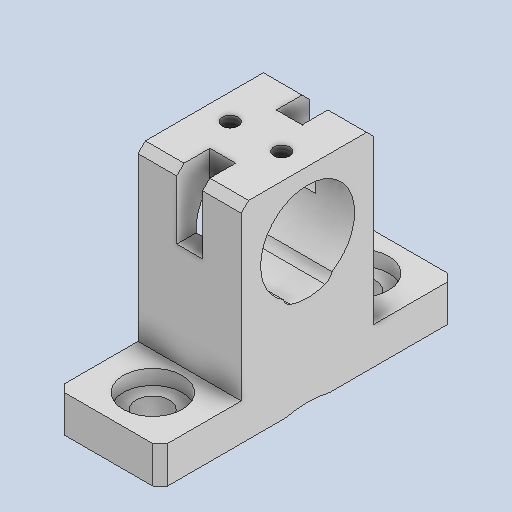
# Autodesk Inventor part: ADAPTER_collimator-BH19.05-D12.7
Saved by Autodesk Inventor 2024.2 (Build 282272000, 272)
## iProperties
Created: 2020-10-22
Part Number: ADAPTER_collimator-BH19.05-D12.7
Material: Generic
Document SubType Name: Modeling
Designer: qiti1
Density: 1 g/cm^3
Appearance: Default
ItemSpecifications: {"_id":"603fbb7ae0b54a000914fb10","finish":"543ef1f380da5b0c476373c1","finish_location":null,"material":"5515e170db035c20ce34af9a","process_initialism":null,"quotes":null,"current_quote":null,"quantity_ordered":1,"features":null,"hardware":null,"threading":null,"part_markings":[],"surface_roughness":null,"tolerance":null,"weld_quantity":null,"Notes":"","certifications":[],"part":null,"revision_num":0,"last_history":null,"inspection_requirement_details":{"inspection_requirement":"std","customer_data_sheet":null},"feedback":null}
Author: qiti1
Autodesk Inventor part; units mm, degrees
note: some values were not read from the file. Chosen so that the rebuilt part matches the saved one: direction of "Hole3".
ref_plane "YZ Plane" through (0, 0, 0) normal (1, 0, 0) x (0, 1, 0)
ref_plane "XZ Plane" through (0, 0, 0) normal (0, 1, 0) x (-1, 0, 0)
ref_plane "XY Plane" through (0, 0, 0) normal (0, 0, 1) x (1, 0, 0)
sketch "Sketch1" plane through (0, 0, 0) normal (0, 1, 0) x (-1, 0, 0)
  line L0 (7, 9) -> (-7, 9)
  line L1 (-7, 9) -> (-7, -9)
  line L2 (-7, -9) -> (7, -9)
  line L3 (7, -9) -> (7, 9)
  line L4 (7, 9) -> (-7, -9) construction
  line L5 (-7, 9) -> (7, -9) construction
  point P0 (0, 0)
  dimension "POST_WIDTH" = 18
  dimension "POST_LENGTH" = 14
  constraints: 12 end point, 2 midpoint, 2 parallel, 1 horizontal, 1 perpendicular
  measures "POST_WIDTH" distance of L2.end L0.start
  measures "POST_LENGTH" distance of L1.end L2.end
extrude "Extrusion1" add sketch "Sketch1" along normal blind 28.05
sketch "Sketch2" plane through (0, 0, 0) normal (0, -1, 0) x (1, 0, 0)
  line L0 (-7, -20) -> (7, -20)
  line L1 (7, -20) -> (7, 20)
  line L2 (7, 20) -> (-7, 20)
  line L3 (-7, 20) -> (-7, -20)
  line L4 (-7, -20) -> (7, 20) construction
  line L5 (7, -20) -> (-7, 20) construction
  line L6 (-7, -9) -> (-7, 9) projected
  line L7 (-7, 9) -> (7, 9) projected
  point P0 (0, 0)
  dimension "d4" = 0
  dimension "d5" = 11
  constraints: 12 end point, 2 midpoint, 2 parallel, 1 horizontal, 1 perpendicular
  measures "d4" distance between parallel lines of L6 L3
  measures "d5" distance between parallel lines of L2 L7
extrude "Extrusion2" add sketch "Sketch2" against normal blind 5
sketch "Sketch3" plane through (0, 5, 0) normal (0, 1, 0) x (1, 0, 0)
  line L0 (-7, 20) -> (7, 20) projected
  line L1 (0, 20) -> (0, -20)
  line L2 (7, -20) -> (-7, -20) projected
  line L3 (7, -9) -> (7, 9) projected
  line L4 (7, 0) -> (-7, 0)
  line L5 (-7, 20) -> (-7, -20) projected
  point P0 (0, 0)
  point P1 (0, -14)
  point P2 (0, 14)
  dimension "d15" = 0
  dimension "d16" = 6
  constraints: 4 end point, 4 midpoint, 1 symmetric about line
  measures "d15" distance from line of L1 point (0, -14)
  measures "d16" distance from line of L2 point (0, -14)
hole "Hole1" at (0, 5, 14) at (0, 5, -14) direction (0, -1, 0) diameter 4.5 end through all counterbore diameter 8 counterbore depth 2 clearance for "Socket Head Cap Screw" size "#8" standard "Ansi Unified Screw Threads"
chamfer "Chamfer2" distance 1 angle 45 2 edges at (0, 28.05, 9) (0, 28.05, -9)
sketch "Sketch8" plane through (7, 5, -9) normal (1, 0, 0) x (0, 0, -1)
  circle A0 centre (-9, 14.4933) radius 6.375
  circle A1 centre (-9, 14.4933) radius 6.883
  circle A2 centre (-10.8329, 9.4575) radius 1.524
  line L0 (-9, 14.4933) -> (-9, 7.6103)
  circle A3 centre (-7.1671, 9.4575) radius 1.524
  line L1 (-9, 14.4933) -> (-10.8329, 9.4575)
  line L2 (-18, 0) -> (-18, 22.05) projected
  line L3 (-17, 23.05) -> (-1, 23.05) projected
  circle A4 centre (-9, 14.05) radius 6
  line L4 (11, -5) -> (-29, -5) projected
  point P0 (-9, -5)
  point P1 (-6.6459, 8.0254)
  point P2 (-8.0195, 8.1942)
  point P3 (-12.2979, 9.0376)
  point P4 (-11.3541, 8.0254)
  point P5 (-5.7021, 9.0376)
  point P6 (-9.9805, 8.1942)
  dimension "d95" = 12
  dimension "HOLE_SIZE" = 12.75
  dimension "THREE_POINT_SIZE" = 13.766
  dimension "d51" = 3.048
  dimension "d52" = 20
  dimension "d55" = 9
  dimension "d96" = 19.05
  constraints: 4 end point, 1 centre point, 1 coincident, 1 point on line, 1 symmetric about line, 1 vertical, 14 other
  measures "d51" diameter of A2
  measures "d52" angle of L0 L1
  measures "d55" distance from line of L2 point (-9, 14.493)
  measures "d96" distance from line of L4 point (-9, 14.05)
extrude "Extrusion6" cut sketch "Sketch8" against normal up to surface (14 mm away) contours A0 A4 | A2 A0 | A4 A3 A0 L0 L1 A2 | A4 A2 | A0 A2 A4 | A4 A3 A0 | A0 A3 | A3 A4 | A2 L1 L0 A0 | A0 L0 A4 A2 | A2 A4 L0 A1 | A3 A4 L0 A0 | A1 L0 A4 A3
sketch "Sketch9" plane through (0, 28.05, 0) normal (0, 1, 0) x (1, 0, 0)
  line L0 (-7, 8) -> (-7, -8) projected
  line L1 (-7, -9) -> (7, -9) projected
  line L2 (7, -8) -> (7, 8) projected
  point P0 (0, 0)
  point P1 (-3.5, 0)
  point P2 (3.5, 0)
  dimension "d64" = 3.5
  dimension "d65" = 9
  dimension "d94" = 3.5
  measures "d64" distance from line of L0 point (-3.5, 0)
  measures "d65" distance from line of L1 point (-3.5, 0)
  measures "d94" distance from line of point (3.5, 0) L2
hole "Hole3" at (-3.5, 28.05, 0) at (3.5, 28.05, 0) direction (0, -1, 0) diameter 2.1565 end up to surface thread size "4-40 UNC" class "2B" standard "ANSI Unified Screw Threads"
chamfer "Chamfer3" distance 1 angle 45 4 edges at (7, 2.5, 20) (-7, 2.5, 20) (7, 2.5, -20) (-7, 2.5, -20)
sketch "Sketch10" plane through (0, 28.05, 0) normal (0, 1, 0) x (1, 0, 0)
  line L0 (-7, -9) -> (7, -9) projected
  line L1 (-1.75, -9) -> (1.75, -9)
  line L2 (1.75, -9) -> (1.75, -4.5)
  line L3 (1.75, -4.5) -> (-1.75, -4.5)
  line L4 (-1.75, -4.5) -> (-1.75, -9)
  line L5 (7, 9) -> (-7, 9) projected
  line L6 (-9.8, 0) -> (9.8, 0) projected
  line L7 (-1.75, 9) -> (1.75, 9)
  line L8 (1.75, 9) -> (1.75, 4.5)
  line L9 (1.75, 4.5) -> (-1.75, 4.5)
  line L10 (-1.75, 4.5) -> (-1.75, 9)
  point P0 (0, 0)
  point P1 (1.75, 5.6664)
  point P2 (1.75, 9)
  dimension "d71" = 4.5
  dimension "d72" = 3.5
  dimension "d73" = 1.75
  constraints: 16 end point, 4 point on line, 3 symmetric about line, 2 parallel, 1 horizontal, 1 perpendicular
  measures "d71" distance between parallel lines of L0 L3
  measures "d72" distance between parallel lines of L2 L4
  measures "d73" distance from line of point (0, 0) L4
extrude "Extrusion7" cut sketch "Sketch10" against normal blind 9
sketch "Sketch11" plane through (0, 0, 0) normal (0, -1, 0) x (1, 0, 0)
  line L0 (0, -4.5) -> (0, -5.5) construction
  line L1 (-1.05, -4.5) -> (-1.05, -5.5)
  line L2 (1.05, -5.5) -> (1.05, -4.5)
  arc A0 (1.05, -4.5) -> (-1.05, -4.5) centre (0, -4.5) ccw
  arc A1 (-1.05, -5.5) -> (1.05, -5.5) centre (0, -5.5) ccw
  point P0 (0, 0)
  point P1 (0, 5)
  point P2 (0, -5)
  dimension "d74" = 10
  dimension "d75" = 0
  dimension "d76" = 0
  dimension "d77" = 5
  dimension "d78" = 1.05
  dimension "d79" = 1
  constraints: 8 end point, 4 point on circle, 4 tangent, 2 centre point, 1 midpoint, 1 parallel, 1 vertical
  measures "d74" distance of point (0, 5) point (0, -5)
  measures "d75" horizontal distance of point (0, -5) point (0, 5)
  measures "d76" horizontal distance of point (0, 0) point (0, 5)
  measures "d77" distance of point (0, 0) point (0, 5)
  measures "d78" radius of A0
  measures "d79" distance of L0.start L0.end
hole "Hole4" at (0, 0, 5) direction (0, 1, 0) diameter 2.1 depth 2.1
extrude "Extrusion8" cut sketch "Sketch11" against normal blind 2.1
sketch "Sketch12" plane through (-7, 5, 9) normal (-1, 0, 0) x (0, 0, 1)
  circle A0 centre (-9, -17.35) radius 12.7
  point P0 (-9, -5)
  dimension "d89" = 0
  dimension "d90" = 12.35
  dimension "d91" = 25.4
  constraints: 1 centre point
  measures "d89" horizontal distance of A0.centre point (-9, -5)
  measures "d90" distance of point (-9, -5) A0.centre
  measures "d91" diameter of A0
extrude "Extrusion9" cut sketch "Sketch12" against normal up to surface (14 mm away)
equation "\"HOLE_SIZE\" = 2 * HOLE_RADIUS + HOLE_TOLERANCE"
equation "\"d52\" = 0.5 * THREE_POINT_ANGLE"
equation "\"d55\" = 0.5 * POST_WIDTH"
equation "\"d96\" = BEAM_HEIGHT"
equation "\"d64\" = 0.25 * POST_LENGTH"
equation "\"d65\" = 0.5 * POST_WIDTH"
equation "\"d94\" = d64"
equation "\"d71\" = 0.25 * POST_WIDTH"
equation "\"d72\" = 0.25 * POST_LENGTH"
equation "\"d73\" = 0.125 * POST_LENGTH"
equation "\"d69\" = EDGE_TO_HOLE"
equation "\"EDGE_TO_HOLE\" = POST_HEIGHT - BEAM_HEIGHT"
equation "\"BEAM_HEIGHT\" = 19.05"
equation "\"COLLIMATOR_DIAMETER\" = 12"
equation "\"THREE_POINT_ANGLE\" = 40deg"
equation "\"HOLE_RADIUS\" = 6.35"
equation "\"HOLE_TOLERANCE\" = 0.05"
equation "\"POST_HEIGHT\" = 28.05"
body "Solid1"
